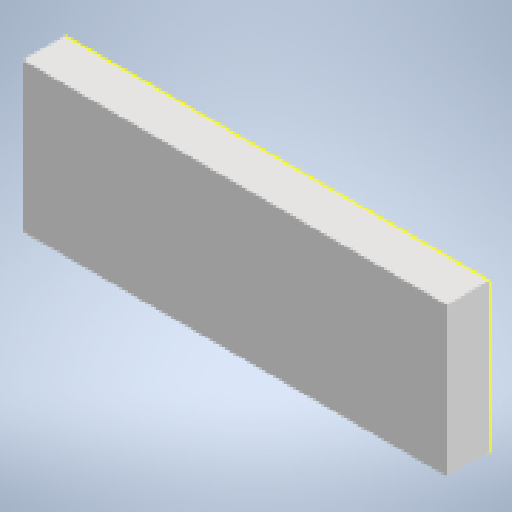
# Autodesk Inventor part: test_izbrisi
Saved by Autodesk Inventor 2023 (Build 270158000, 158)
## iProperties
Created: 2022-09-28
Part Number: test_izbrisi
Material: Generic
Document SubType Name: Modeling
Designer: simon
Density: 1 g/cm^3
Appearance: Default
Author: simon
Autodesk Inventor part; units mm, degrees
ref_plane "YZ Plane" through (0, 0, 0) normal (1, 0, 0) x (0, 1, 0)
ref_plane "XZ Plane" through (0, 0, 0) normal (0, 1, 0) x (-1, 0, 0)
ref_plane "XY Plane" through (0, 0, 0) normal (0, 0, 1) x (1, 0, 0)
sketch "Sketch5" plane through (0, 0, 0) normal (0, 0, 1) x (1, 0, 0)
  line L0 (7, -1.5) -> (0.5048, -1.5) projected
  circle A0 centre (14.7, 0) radius 1.25 projected
  circle A1 centre (-0.7, 0) radius 1.25 projected
  line L1 (-3, -3.5) -> (17, -3.5) projected
  line L2 (17, -3.5) -> (17, 3.5) projected
  line L3 (17, 3.5) -> (-3, 3.5) projected
  line L4 (-3, 3.5) -> (-3, -3.5) projected
  point P0 (0, 0)
extrude "Extrusion7" add sketch "Sketch5" along normal blind 2 contours A0 | A1 | L4 L3 L2 L1
extrude "Extrusion8" add sketch "Sketch5" against normal blind 2 contours A0 | A1
body "Solid4"
